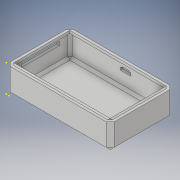
# Autodesk Inventor part: Base
Saved by Autodesk Inventor 2019 (Build 230136000, 136)
## iProperties
Created: 2021-04-26
Part Number: Base
Material: Všeobecné
Document SubType Name: Modeling
Designer: miko flosso
Density: 1 g/cm^3
Appearance: Výchozí
Author: miko flosso
Autodesk Inventor part; units mm, degrees
ref_plane "YZ Plane" through (0, 0, 0) normal (1, 0, 0) x (0, 1, 0)
ref_plane "XZ Plane" through (0, 0, 0) normal (0, 1, 0) x (-1, 0, 0)
ref_plane "XY Plane" through (0, 0, 0) normal (0, 0, 1) x (1, 0, 0)
sketch "Náčrt1" plane through (0, 0, 0) normal (0, 1, 0) x (-1, 0, 0)
  line L0 (0, 0) -> (-80, 0)
  line L1 (-80, 0) -> (-80, -49)
  line L2 (-80, -49) -> (0, -49)
  line L3 (0, -49) -> (0, 0)
  dimension "d0" = 80
  dimension "d1" = 49
  constraints: 8 end point, 2 parallel, 1 horizontal, 1 perpendicular
  measures "d0" distance of L2.end L1.end
  measures "d1" distance of L1.end L0.end
extrude "Vysunutí1" add sketch "Náčrt1" along normal blind 20
chamfer "Zkosení1" distance 3 angle 45 7 edges at (80, 10, 0) (40, 0, 0) (0, 0, -24.5) (0, 10, -49) (80, 10, -49) (40, 0, -49) (80, 0, -24.5)
chamfer "Zkosení2" distance 3 angle 45 1 edges at (0, 11.5, 0)
shell "Skořepina1" thickness 2 removed faces 1 at (27.6667, 20, -32.6667)
sketch "Náčrt2" plane through (0, 3, -46) normal (-1, 0, 0) x (0, 0, 1)
  line L0 (7, 14) -> (36, 14)
  line L1 (36, 14) -> (36, 11)
  line L2 (36, 11) -> (7, 11)
  line L3 (7, 11) -> (7, 14)
  line L4 (0, 0) -> (0, 17) projected
  line L5 (0, -3) -> (43, -3) projected
  line L6 (43, 0) -> (0, 0) projected
  line L7 (0, 17) -> (43, 17) projected
  point P0 (46, -3)
  dimension "d11" = 29
  dimension "d12" = 3
  dimension "d13" = 7
  dimension "d17" = 3
  constraints: 8 end point, 2 parallel, 1 horizontal, 1 perpendicular
  measures "d11" distance of L1.end L2.end
  measures "d12" distance of L0.end L1.end
  measures "d13" distance between parallel lines of L4 L3
  measures "d17" distance between parallel lines of L7 L0
extrude "Vysunutí2" cut sketch "Náčrt2" against normal blind 2.5
sketch "Náčrt3" plane through (0, 14, -39) normal (0, 0, 1) x (1, 0, 0)
  point P0 (0, -14)
sketch "Náčrt4" plane through (77, 3, -49) normal (0, 0, -1) x (-1, 0, 0)
  line L0 (28, 13) -> (36, 13)
  line L1 (36, 13) -> (36, 10)
  line L2 (36, 10) -> (28, 10)
  line L3 (28, 10) -> (28, 13)
  line L4 (0, 0) -> (0, 17) projected
  line L5 (74, 0) -> (0, 0) projected
  point P0 (77, -3)
  dimension "d20" = 8
  dimension "d21" = 3
  dimension "d22" = 28
  dimension "d23" = 10
  constraints: 8 end point, 2 parallel, 1 horizontal, 1 perpendicular
  measures "d20" distance of L1.end L2.end
  measures "d21" distance of L0.end L1.end
  measures "d22" distance between parallel lines of L3 L4
  measures "d23" distance between parallel lines of L5 L2
extrude "Vysunutí3" cut sketch "Náčrt4" against normal blind 2.5
chamfer "Zkosení3" distance 1 angle 60 1 edges at (49, 16, -48) measured on face at (49, 15.5, -48)
chamfer "Zkosení4" distance 1 angle 60 1 edges at (41, 16, -48) measured on face at (41, 15.5, -48)
sketch "Náčrt5" plane through (77, 3, 0) normal (0, 0, 1) x (1, 0, 0)
  point P0 (-77, -3)
sketch "Náčrt6" plane through (77, 3, -49) normal (0, 0, -1) x (-1, 0, 0)
  point P0 (77, -3)
sketch "Náčrt7" plane through (2, 3.8284, -3.8284) normal (1, 0, 0) x (0, 0, -1)
  point P0 (-3.8284, -3.8284)
sketch "Náčrt8" plane through (0, 20, 0) normal (0, 1, 0) x (1, 0, 0)
  line L0 (2, 3.8284) -> (2, 45.1716) projected
  line L1 (2, 3.8284) -> (2, 45.1716)
  line L2 (3.8284, 47) -> (76.1716, 47) projected
  line L3 (2, 45.1716) -> (3.8284, 47)
  line L4 (3.8284, 47) -> (76.1716, 47)
  line L5 (76.1716, 47) -> (78, 45.1716)
  line L6 (78, 45.1716) -> (78, 3.8284) projected
  line L7 (78, 45.1716) -> (78, 3.8284)
  line L8 (78, 3.8284) -> (76.1716, 2)
  line L9 (76.1716, 2) -> (3.8284, 2)
  line L10 (3.8284, 2) -> (2, 3.8284)
  point P0 (0, 0)
  constraints: 16 end point, 4 equal length, 3 perpendicular
extrude "Vysunutí4" add sketch "Náčrt8" along normal mid plane 2
sketch "Náčrt9" plane through (0, 21, 0) normal (0, 1, 0) x (1, 0, 0)
  point P0 (0, 0)
chamfer "Zkosení5" distance 1 angle 45 4 edges at (40, 21, -2) (78, 21, -24.5) (40, 21, -47) (2, 21, -24.5)
sketch "Náčrt10" plane through (0, 21, 0) normal (0, 1, 0) x (1, 0, 0)
  point P0 (0, 0)
sketch "Náčrt11" plane through (0, 21, 0) normal (0, 1, 0) x (1, 0, 0)
  line L0 (3, 46) -> (77, 46) projected
  line L1 (76.1716, 2) -> (78, 3.8284) projected
  line L2 (3, 46) -> (77.0858, 46)
  line L3 (77.0858, 46) -> (77.0858, 2.9142)
  line L4 (77.0858, 2.9142) -> (3, 2.9142)
  line L5 (3, 2.9142) -> (3, 46)
  point P0 (0, 0)
  constraints: 8 end point, 2 parallel, 1 horizontal, 1 midpoint, 1 perpendicular
extrude "Vysunutí5" cut sketch "Náčrt11" against normal blind 5
